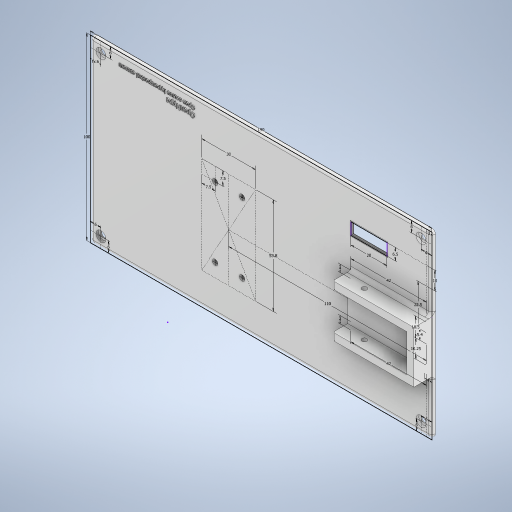
# Autodesk Inventor part: BoxCover
Saved by Autodesk Inventor 2023 (Build 270158000, 158)
## iProperties
Created: 2022-10-22
Part Number: BoxCover
Material: ABS Plastic
Document SubType Name: Modeling
Designer: Miner
Density: 1.06 g/cm^3
Appearance: Smooth - White
Author: Miner
Autodesk Inventor part; units mm, degrees
(part 1 of 2)
ref_plane "YZ Plane" through (0, 0, 0) normal (1, 0, 0) x (0, 1, 0)
ref_plane "XZ Plane" through (0, 0, 0) normal (0, 1, 0) x (-1, 0, 0)
ref_plane "XY Plane" through (0, 0, 0) normal (0, 0, 1) x (1, 0, 0)
sketch "Sketch1" plane through (0, 0, 0) normal (0, 0, 1) x (1, 0, 0)
  line L0 (0, 0) -> (-190, 0)
  line L1 (-190, 0) -> (-190, 100)
  line L2 (-190, 100) -> (0, 100)
  line L3 (0, 100) -> (0, 0)
  line L4 (0, 100) -> (-3, 100) construction
  line L5 (-3, 100) -> (-3, 0) construction
  line L6 (-3, 50) -> (-3, 44.6) construction
  line L7 (-3, 44.6) -> (-37.3438, 44.6) construction
  line L8 (-3, 44.6) -> (-3, 34.35) construction
  line L9 (-3, 34.35) -> (-45, 34.35)
  line L10 (-45, 34.35) -> (-45, 30.35)
  line L11 (-45, 30.35) -> (-3, 30.35)
  line L12 (-3, 30.35) -> (-3, 34.35)
  line L13 (-3, 44.6) -> (-3, 55.1) construction
  line L14 (-3, 55.1) -> (-45, 55.1)
  line L15 (-45, 55.1) -> (-45, 59.1)
  line L16 (-45, 59.1) -> (-3, 59.1)
  line L17 (-3, 59.1) -> (-3, 55.1)
  line L18 (0, 59.1) -> (-4, 59.1)
  line L19 (-4, 59.1) -> (-4, 30.35)
  line L20 (-4, 30.35) -> (0, 30.35)
  line L21 (0, 30.35) -> (0, 59.1)
  line L22 (-3, 44.6) -> (-113, 44.6) construction
  line L23 (-128, 17.7) -> (-98, 17.7) construction
  line L24 (-98, 17.7) -> (-98, 71.5) construction
  line L25 (-98, 71.5) -> (-128, 71.5) construction
  line L26 (-128, 71.5) -> (-128, 17.7) construction
  line L27 (-128, 17.7) -> (-98, 71.5) construction
  line L28 (-98, 17.7) -> (-128, 71.5) construction
  line L29 (-128, 71.5) -> (-120.5, 71.5) construction
  line L30 (-120.5, 71.5) -> (-120.5, 64) construction
  line L31 (-120.5, 64) -> (-128, 64) construction
  line L32 (-128, 64) -> (-128, 71.5) construction
  line L33 (-113, 71.5) -> (-113, 17.7) construction
  line L34 (-190, 100) -> (-184, 100) construction
  line L35 (-184, 100) -> (-184, 94) construction
  line L36 (-184, 94) -> (-190, 94) construction
  line L37 (-190, 94) -> (-190, 100) construction
  line L38 (0, 100) -> (-6, 100) construction
  line L39 (-6, 100) -> (-6, 94) construction
  line L40 (-6, 94) -> (0, 94) construction
  line L41 (0, 94) -> (0, 100) construction
  line L42 (0, 0) -> (-6, 0) construction
  line L43 (-6, 0) -> (-6, 6) construction
  line L44 (-6, 6) -> (0, 6) construction
  line L45 (0, 6) -> (0, 0) construction
  line L46 (-190, 0) -> (-184, 0) construction
  line L47 (-184, 0) -> (-184, 6) construction
  line L48 (-184, 6) -> (-190, 6) construction
  line L49 (-190, 6) -> (-190, 0) construction
  line L50 (-4, 55.1) -> (-45, 55.1)
  line L51 (-45, 55.1) -> (-45, 34.35)
  line L52 (-45, 34.35) -> (-4, 34.35)
  line L53 (-4, 34.35) -> (-4, 55.1)
  line L54 (-3, 50) -> (-3, 72.5) construction
  line L55 (-3, 72.5) -> (-3, 82.5) construction
  line L56 (-3, 82.5) -> (-45, 82.5) construction
  line L57 (-45, 82.5) -> (-25, 82.5) construction
  line L58 (-25, 82.5) -> (-25, 76)
  line L59 (-25, 76) -> (-45, 76)
  line L60 (-45, 76) -> (-45, 82.5)
  line L61 (-45, 82.5) -> (-25, 82.5)
  line L62 (-131.617, 88.8001) -> (-198.0641, 88.8001) construction
  line L63 (-198.0641, 88.8001) -> (-198.0641, 103.0152) construction
  line L64 (-198.0641, 103.0152) -> (-131.617, 103.0152) construction
  line L65 (-131.617, 103.0152) -> (-131.617, 88.8001) construction
  spline S0 degree 2 poles (-133.6389, 89.1384) (-133.7807, 89.3045) (-133.9387, 89.7908) (-133.9387, 90.1028) knots 0 0 0 1 2 2 2
  spline S1 degree 2 poles (-133.9387, 90.1028) (-133.9387, 90.4066) (-133.7847, 90.899) (-133.6389, 91.0651) knots 0 0 0 1 2 2 2
  spline S2 degree 2 poles (-133.6389, 91.0651) (-133.4849, 91.2393) (-133.0777, 91.4054) (-132.8326, 91.4054) knots 0 0 0 1 2 2 2
  spline S3 degree 2 poles (-132.8326, 91.4054) (-132.5793, 91.4054) (-132.1741, 91.2332) (-132.0262, 91.0651) knots 0 0 0 1 2 2 2
  spline S4 degree 2 poles (-132.0262, 91.0651) (-131.8824, 90.899) (-131.7284, 90.4107) (-131.7284, 90.1028) knots 0 0 0 1 2 2 2
  spline S5 degree 2 poles (-131.7284, 90.1028) (-131.7284, 89.7887) (-131.8844, 89.3106) (-132.0283, 89.1384) knots 0 0 0 1 2 2 2
  spline S6 degree 2 poles (-132.0283, 89.1384) (-132.1741, 88.9723) (-132.5813, 88.8001) (-132.8326, 88.8001) knots 0 0 0 1 2 2 2
  spline S7 degree 2 poles (-132.8326, 88.8001) (-133.0878, 88.8001) (-133.4971, 88.9784) (-133.6389, 89.1384) knots 0 0 0 1 2 2 2
  spline S8 degree 2 poles (-133.5923, 90.1028) (-133.5923, 89.8556) (-133.4849, 89.4727) (-133.3877, 89.3471) knots 0 0 0 1 2 2 2
  spline S9 degree 2 poles (-133.3877, 89.3471) (-133.2884, 89.2174) (-133.0088, 89.0878) (-132.8346, 89.0878) knots 0 0 0 1 2 2 2
  spline S10 degree 2 poles (-132.8346, 89.0878) (-132.6543, 89.0878) (-132.3828, 89.2134) (-132.2795, 89.3471) knots 0 0 0 1 2 2 2
  spline S11 degree 2 poles (-132.2795, 89.3471) (-132.1802, 89.4747) (-132.0749, 89.8596) (-132.0749, 90.1028) knots 0 0 0 1 2 2 2
  spline S12 degree 2 poles (-132.0749, 90.1028) (-132.0749, 90.5951) (-132.4881, 91.1178) (-132.8346, 91.1178) knots 0 0 0 1 2 2 2
  spline S13 degree 2 poles (-132.8346, 91.1178) (-133.181, 91.1178) (-133.5923, 90.5951) (-133.5923, 90.1028) knots 0 0 0 1 2 2 2
  spline S14 degree 2 poles (-135.8512, 90.3641) (-135.8512, 90.8341) (-135.4035, 91.3892) (-135.0611, 91.3892) knots 0 0 0 1 2 2 2
  spline S15 degree 2 poles (-135.0611, 91.3892) (-134.9213, 91.3892) (-134.7065, 91.3244) (-134.5951, 91.2575) knots 0 0 0 1 2 2 2
  line L66 (-134.5951, 91.2575) -> (-134.5951, 92.0436)
  line L67 (-134.5951, 92.0436) -> (-134.2791, 92.0436)
  line L68 (-134.2791, 92.0436) -> (-134.2791, 89.4767)
  line L69 (-134.2791, 89.4767) -> (-134.5951, 89.4767)
  line L70 (-134.5951, 89.4767) -> (-134.5951, 89.6733)
  spline S16 degree 2 poles (-134.5951, 89.6733) (-134.7126, 89.5659) (-135.0003, 89.4241) (-135.1685, 89.4241) knots 0 0 0 1 2 2 2
  spline S17 degree 2 poles (-135.1685, 89.4241) (-135.4906, 89.4241) (-135.8512, 89.9346) (-135.8512, 90.3641) knots 0 0 0 1 2 2 2
  spline S18 degree 2 poles (-135.525, 90.4006) (-135.525, 90.0784) (-135.3204, 89.7239) (-135.0915, 89.7239) knots 0 0 0 1 2 2 2
  spline S19 degree 2 poles (-135.0915, 89.7239) (-134.9578, 89.7239) (-134.7065, 89.8434) (-134.5951, 89.9366) knots 0 0 0 1 2 2 2
  line L71 (-134.5951, 89.9366) -> (-134.5951, 91.0023)
  spline S20 degree 2 poles (-134.5951, 91.0023) (-134.7187, 91.061) (-134.895, 91.1056) (-135.0084, 91.1056) knots 0 0 0 1 2 2 2
  spline S21 degree 2 poles (-135.0084, 91.1056) (-135.2535, 91.1056) (-135.525, 90.745) (-135.525, 90.4006) knots 0 0 0 1 2 2 2
  spline S22 degree 2 poles (-136.9938, 91.3953) (-136.5441, 91.3953) (-136.0497, 90.8908) (-136.0497, 90.4249) knots 0 0 0 1 2 2 2
  spline S23 degree 2 poles (-136.0497, 90.4249) (-136.0497, 89.967) (-136.5299, 89.4241) (-136.9168, 89.4241) knots 0 0 0 1 2 2 2
  spline S24 degree 2 poles (-136.9168, 89.4241) (-137.0911, 89.4241) (-137.3605, 89.5254) (-137.4598, 89.6327) knots 0 0 0 1 2 2 2
  spline S25 degree 2 poles (-137.4598, 89.6327) (-137.5611, 89.7401) (-137.6685, 90.0501) (-137.6685, 90.275) knots 0 0 0 1 2 2 2
  line L72 (-137.6685, 90.275) -> (-137.6685, 90.4472)
  line L73 (-137.6685, 90.4472) -> (-136.3698, 90.4472)
  spline S26 degree 2 poles (-136.3698, 90.4472) (-136.3698, 90.7733) (-136.698, 91.1198) (-136.9898, 91.1198) knots 0 0 0 1 2 2 2
  spline S27 degree 2 poles (-136.9898, 91.1198) (-137.0931, 91.1198) (-137.2937, 91.0732) (-137.3747, 91.0367) knots 0 0 0 1 2 2 2
  spline S28 degree 2 poles (-137.3747, 91.0367) (-137.4598, 90.9962) (-137.5773, 90.9253) (-137.6158, 90.8929) knots 0 0 0 1 2 2 2
  line L74 (-137.6158, 90.8929) -> (-137.634, 90.8929)
  line L75 (-137.634, 90.8929) -> (-137.634, 91.2373)
  spline S29 degree 2 poles (-137.634, 91.2373) (-137.5793, 91.2596) (-137.4132, 91.3244) (-137.3484, 91.3426) knots 0 0 0 1 2 2 2
  spline S30 degree 2 poles (-137.3484, 91.3426) (-137.2572, 91.369) (-137.1073, 91.3953) (-136.9938, 91.3953) knots 0 0 0 1 2 2 2
  spline S31 degree 2 poles (-137.3605, 90.2061) (-137.3565, 90.0784) (-137.3038, 89.8921) (-137.2531, 89.8293) knots 0 0 0 1 2 2 2
  spline S32 degree 2 poles (-137.2531, 89.8293) (-137.1984, 89.7584) (-137.0262, 89.6834) (-136.8986, 89.6834) knots 0 0 0 1 2 2 2
  spline S33 degree 2 poles (-136.8986, 89.6834) (-136.773, 89.6834) (-136.5967, 89.7584) (-136.5238, 89.8313) knots 0 0 0 1 2 2 2
  spline S34 degree 2 poles (-136.5238, 89.8313) (-136.4529, 89.9062) (-136.38, 90.0866) (-136.3698, 90.2061) knots 0 0 0 1 2 2 2
  line L76 (-136.3698, 90.2061) -> (-137.3605, 90.2061)
  line L77 (-139.4614, 91.3528) -> (-139.1454, 91.3528)
  line L78 (-139.1454, 91.3528) -> (-139.1454, 90.2831)
  spline S35 degree 2 poles (-139.1454, 90.2831) (-139.1454, 90.1534) (-139.121, 89.9306) (-139.0846, 89.8637) knots 0 0 0 1 2 2 2
  spline S36 degree 2 poles (-139.0846, 89.8637) (-139.0461, 89.7928) (-138.9083, 89.7239) (-138.7908, 89.7239) knots 0 0 0 1 2 2 2
  spline S37 degree 2 poles (-138.7908, 89.7239) (-138.6733, 89.7239) (-138.4241, 89.8495) (-138.3046, 89.9508) knots 0 0 0 1 2 2 2
  line L79 (-138.3046, 89.9508) -> (-138.3046, 91.3528)
  line L80 (-138.3046, 91.3528) -> (-137.9885, 91.3528)
  line L81 (-137.9885, 91.3528) -> (-137.9885, 89.4767)
  line L82 (-137.9885, 89.4767) -> (-138.3046, 89.4767)
  line L83 (-138.3046, 89.4767) -> (-138.3046, 89.6854)
  spline S38 degree 2 poles (-138.3046, 89.6854) (-138.4464, 89.5578) (-138.7199, 89.4241) (-138.8739, 89.4241) knots 0 0 0 1 2 2 2
  spline S39 degree 2 poles (-138.8739, 89.4241) (-139.1494, 89.4241) (-139.4614, 89.7887) (-139.4614, 90.1352) knots 0 0 0 1 2 2 2
  line L84 (-139.4614, 90.1352) -> (-139.4614, 91.3528)
  line L85 (-141.7446, 91.3528) -> (-141.4124, 91.3528)
  line L86 (-141.4124, 91.3528) -> (-141.4124, 90.1291)
  line L87 (-141.4124, 90.1291) -> (-140.2616, 90.1291)
  line L88 (-140.2616, 90.1291) -> (-140.2616, 91.3528)
  line L89 (-140.2616, 91.3528) -> (-139.9294, 91.3528)
  line L90 (-139.9294, 91.3528) -> (-139.9294, 88.8528)
  line L91 (-139.9294, 88.8528) -> (-140.2616, 88.8528)
  line L92 (-140.2616, 88.8528) -> (-140.2616, 89.8333)
  line L93 (-140.2616, 89.8333) -> (-141.4124, 89.8333)
  line L94 (-141.4124, 89.8333) -> (-141.4124, 88.8528)
  line L95 (-141.4124, 88.8528) -> (-141.7446, 88.8528)
  line L96 (-141.7446, 88.8528) -> (-141.7446, 91.3528)
  line L97 (-143.6997, 89.4767) -> (-142.6907, 92.0436)
  line L98 (-142.6907, 92.0436) -> (-142.3524, 92.0436)
  line L99 (-142.3524, 92.0436) -> (-142.6887, 91.2616)
  line L100 (-142.6887, 91.2616) -> (-142.008, 89.4767)
  line L101 (-142.008, 89.4767) -> (-142.3484, 89.4767)
  line L102 (-142.3484, 89.4767) -> (-142.8609, 90.8665)
  line L103 (-142.8609, 90.8665) -> (-143.3714, 89.4767)
  line L104 (-143.3714, 89.4767) -> (-143.6997, 89.4767)
  spline S40 degree 2 poles (-145.5108, 90.3641) (-145.5108, 90.8341) (-145.0631, 91.3892) (-144.7207, 91.3892) knots 0 0 0 1 2 2 2
  spline S41 degree 2 poles (-144.7207, 91.3892) (-144.5809, 91.3892) (-144.3662, 91.3244) (-144.2548, 91.2575) knots 0 0 0 1 2 2 2
  line L105 (-144.2548, 91.2575) -> (-144.2548, 92.0436)
  line L106 (-144.2548, 92.0436) -> (-143.9387, 92.0436)
  line L107 (-143.9387, 92.0436) -> (-143.9387, 89.4767)
  line L108 (-143.9387, 89.4767) -> (-144.2548, 89.4767)
  line L109 (-144.2548, 89.4767) -> (-144.2548, 89.6733)
  spline S42 degree 2 poles (-144.2548, 89.6733) (-144.3723, 89.5659) (-144.6599, 89.4241) (-144.8281, 89.4241) knots 0 0 0 1 2 2 2
  spline S43 degree 2 poles (-144.8281, 89.4241) (-145.1502, 89.4241) (-145.5108, 89.9346) (-145.5108, 90.3641) knots 0 0 0 1 2 2 2
  spline S44 degree 2 poles (-145.1847, 90.4006) (-145.1847, 90.0784) (-144.98, 89.7239) (-144.7511, 89.7239) knots 0 0 0 1 2 2 2
  spline S45 degree 2 poles (-144.7511, 89.7239) (-144.6174, 89.7239) (-144.3662, 89.8434) (-144.2548, 89.9366) knots 0 0 0 1 2 2 2
  line L110 (-144.2548, 89.9366) -> (-144.2548, 91.0023)
  spline S46 degree 2 poles (-144.2548, 91.0023) (-144.3783, 91.061) (-144.5546, 91.1056) (-144.668, 91.1056) knots 0 0 0 1 2 2 2
  spline S47 degree 2 poles (-144.668, 91.1056) (-144.9132, 91.1056) (-145.1847, 90.745) (-145.1847, 90.4006) knots 0 0 0 1 2 2 2
  spline S48 degree 2 poles (-146.6535, 91.3953) (-146.2037, 91.3953) (-145.7094, 90.8908) (-145.7094, 90.4249) knots 0 0 0 1 2 2 2
  spline S49 degree 2 poles (-145.7094, 90.4249) (-145.7094, 89.967) (-146.1895, 89.4241) (-146.5765, 89.4241) knots 0 0 0 1 2 2 2
  spline S50 degree 2 poles (-146.5765, 89.4241) (-146.7507, 89.4241) (-147.0202, 89.5254) (-147.1194, 89.6327) knots 0 0 0 1 2 2 2
  spline S51 degree 2 poles (-147.1194, 89.6327) (-147.2207, 89.7401) (-147.3281, 90.0501) (-147.3281, 90.275) knots 0 0 0 1 2 2 2
  line L111 (-147.3281, 90.275) -> (-147.3281, 90.4472)
  line L112 (-147.3281, 90.4472) -> (-146.0295, 90.4472)
  spline S52 degree 2 poles (-146.0295, 90.4472) (-146.0295, 90.7733) (-146.3577, 91.1198) (-146.6494, 91.1198) knots 0 0 0 1 2 2 2
  spline S53 degree 2 poles (-146.6494, 91.1198) (-146.7527, 91.1198) (-146.9533, 91.0732) (-147.0343, 91.0367) knots 0 0 0 1 2 2 2
  spline S54 degree 2 poles (-147.0343, 91.0367) (-147.1194, 90.9962) (-147.2369, 90.9253) (-147.2754, 90.8929) knots 0 0 0 1 2 2 2
  line L113 (-147.2754, 90.8929) -> (-147.2937, 90.8929)
  line L114 (-147.2937, 90.8929) -> (-147.2937, 91.2373)
  spline S55 degree 2 poles (-147.2937, 91.2373) (-147.239, 91.2596) (-147.0728, 91.3244) (-147.008, 91.3426) knots 0 0 0 1 2 2 2
  spline S56 degree 2 poles (-147.008, 91.3426) (-146.9168, 91.369) (-146.7669, 91.3953) (-146.6535, 91.3953) knots 0 0 0 1 2 2 2
  spline S57 degree 2 poles (-147.0202, 90.2061) (-147.0161, 90.0784) (-146.9634, 89.8921) (-146.9128, 89.8293) knots 0 0 0 1 2 2 2
  spline S58 degree 2 poles (-146.9128, 89.8293) (-146.8581, 89.7584) (-146.6859, 89.6834) (-146.5582, 89.6834) knots 0 0 0 1 2 2 2
  spline S59 degree 2 poles (-146.5582, 89.6834) (-146.4326, 89.6834) (-146.2564, 89.7584) (-146.1834, 89.8313) knots 0 0 0 1 2 2 2
  spline S60 degree 2 poles (-146.1834, 89.8313) (-146.1125, 89.9062) (-146.0396, 90.0866) (-146.0295, 90.2061) knots 0 0 0 1 2 2 2
  line L115 (-146.0295, 90.2061) -> (-147.0202, 90.2061)
  spline S61 degree 2 poles (-133.2345, 93.0672) (-133.3479, 93.2001) (-133.4744, 93.5891) (-133.4744, 93.8387) knots 0 0 0 1 2 2 2
  spline S62 degree 2 poles (-133.4744, 93.8387) (-133.4744, 94.0818) (-133.3512, 94.4756) (-133.2345, 94.6085) knots 0 0 0 1 2 2 2
  spline S63 degree 2 poles (-133.2345, 94.6085) (-133.1113, 94.7479) (-132.7856, 94.8808) (-132.5894, 94.8808) knots 0 0 0 1 2 2 2
  spline S64 degree 2 poles (-132.5894, 94.8808) (-132.3868, 94.8808) (-132.0627, 94.743) (-131.9444, 94.6085) knots 0 0 0 1 2 2 2
  spline S65 degree 2 poles (-131.9444, 94.6085) (-131.8293, 94.4756) (-131.7061, 94.085) (-131.7061, 93.8387) knots 0 0 0 1 2 2 2
  spline S66 degree 2 poles (-131.7061, 93.8387) (-131.7061, 93.5874) (-131.8309, 93.2049) (-131.946, 93.0672) knots 0 0 0 1 2 2 2
  spline S67 degree 2 poles (-131.946, 93.0672) (-132.0627, 92.9343) (-132.3885, 92.7965) (-132.5894, 92.7965) knots 0 0 0 1 2 2 2
  spline S68 degree 2 poles (-132.5894, 92.7965) (-132.7937, 92.7965) (-133.121, 92.9391) (-133.2345, 93.0672) knots 0 0 0 1 2 2 2
  spline S69 degree 2 poles (-133.1972, 93.8387) (-133.1972, 93.6409) (-133.1113, 93.3346) (-133.0335, 93.2341) knots 0 0 0 1 2 2 2
  spline S70 degree 2 poles (-133.0335, 93.2341) (-132.9541, 93.1304) (-132.7304, 93.0267) (-132.5911, 93.0267) knots 0 0 0 1 2 2 2
  spline S71 degree 2 poles (-132.5911, 93.0267) (-132.4468, 93.0267) (-132.2296, 93.1271) (-132.147, 93.2341) knots 0 0 0 1 2 2 2
  spline S72 degree 2 poles (-132.147, 93.2341) (-132.0676, 93.3362) (-131.9833, 93.6442) (-131.9833, 93.8387) knots 0 0 0 1 2 2 2
  spline S73 degree 2 poles (-131.9833, 93.8387) (-131.9833, 94.2325) (-132.3139, 94.6506) (-132.5911, 94.6506) knots 0 0 0 1 2 2 2
  spline S74 degree 2 poles (-132.5911, 94.6506) (-132.8682, 94.6506) (-133.1972, 94.2325) (-133.1972, 93.8387) knots 0 0 0 1 2 2 2
  spline S75 degree 2 poles (-135.0044, 94.0477) (-135.0044, 94.4237) (-134.6462, 94.8678) (-134.3723, 94.8678) knots 0 0 0 1 2 2 2
  spline S76 degree 2 poles (-134.3723, 94.8678) (-134.2604, 94.8678) (-134.0886, 94.816) (-133.9995, 94.7625) knots 0 0 0 1 2 2 2
  line L116 (-133.9995, 94.7625) -> (-133.9995, 95.3913)
  line L117 (-133.9995, 95.3913) -> (-133.7467, 95.3913)
  line L118 (-133.7467, 95.3913) -> (-133.7467, 93.3378)
  line L119 (-133.7467, 93.3378) -> (-133.9995, 93.3378)
  line L120 (-133.9995, 93.3378) -> (-133.9995, 93.4951)
  spline S77 degree 2 poles (-133.9995, 93.4951) (-134.0935, 93.4092) (-134.3236, 93.2957) (-134.4582, 93.2957) knots 0 0 0 1 2 2 2
  spline S78 degree 2 poles (-134.4582, 93.2957) (-134.7159, 93.2957) (-135.0044, 93.7041) (-135.0044, 94.0477) knots 0 0 0 1 2 2 2
  spline S79 degree 2 poles (-134.7434, 94.0769) (-134.7434, 93.8192) (-134.5797, 93.5356) (-134.3966, 93.5356) knots 0 0 0 1 2 2 2
  spline S80 degree 2 poles (-134.3966, 93.5356) (-134.2896, 93.5356) (-134.0886, 93.6312) (-133.9995, 93.7058) knots 0 0 0 1 2 2 2
  line L121 (-133.9995, 93.7058) -> (-133.9995, 94.5583)
  spline S81 degree 2 poles (-133.9995, 94.5583) (-134.0984, 94.6053) (-134.2394, 94.6409) (-134.3301, 94.6409) knots 0 0 0 1 2 2 2
  spline S82 degree 2 poles (-134.3301, 94.6409) (-134.5262, 94.6409) (-134.7434, 94.3524) (-134.7434, 94.0769) knots 0 0 0 1 2 2 2
  spline S83 degree 2 poles (-135.9185, 94.8727) (-135.5586, 94.8727) (-135.1632, 94.4691) (-135.1632, 94.0964) knots 0 0 0 1 2 2 2
  spline S84 degree 2 poles (-135.1632, 94.0964) (-135.1632, 93.7301) (-135.5473, 93.2957) (-135.8569, 93.2957) knots 0 0 0 1 2 2 2
  spline S85 degree 2 poles (-135.8569, 93.2957) (-135.9962, 93.2957) (-136.2118, 93.3767) (-136.2912, 93.4626) knots 0 0 0 1 2 2 2
  spline S86 degree 2 poles (-136.2912, 93.4626) (-136.3723, 93.5485) (-136.4582, 93.7965) (-136.4582, 93.9764) knots 0 0 0 1 2 2 2
  line L122 (-136.4582, 93.9764) -> (-136.4582, 94.1142)
  line L123 (-136.4582, 94.1142) -> (-135.4193, 94.1142)
  spline S87 degree 2 poles (-135.4193, 94.1142) (-135.4193, 94.3751) (-135.6818, 94.6523) (-135.9152, 94.6523) knots 0 0 0 1 2 2 2
  spline S88 degree 2 poles (-135.9152, 94.6523) (-135.9979, 94.6523) (-136.1583, 94.615) (-136.2232, 94.5858) knots 0 0 0 1 2 2 2
  spline S89 degree 2 poles (-136.2232, 94.5858) (-136.2912, 94.5534) (-136.3852, 94.4967) (-136.416, 94.4707) knots 0 0 0 1 2 2 2
  line L124 (-136.416, 94.4707) -> (-136.4306, 94.4707)
  line L125 (-136.4306, 94.4707) -> (-136.4306, 94.7463)
  spline S90 degree 2 poles (-136.4306, 94.7463) (-136.3868, 94.7641) (-136.2539, 94.816) (-136.2021, 94.8306) knots 0 0 0 1 2 2 2
  spline S91 degree 2 poles (-136.2021, 94.8306) (-136.1291, 94.8516) (-136.0092, 94.8727) (-135.9185, 94.8727) knots 0 0 0 1 2 2 2
  spline S92 degree 2 poles (-136.2118, 93.9213) (-136.2086, 93.8192) (-136.1664, 93.6701) (-136.1259, 93.6199) knots 0 0 0 1 2 2 2
  spline S93 degree 2 poles (-136.1259, 93.6199) (-136.0821, 93.5631) (-135.9444, 93.5032) (-135.8423, 93.5032) knots 0 0 0 1 2 2 2
  spline S94 degree 2 poles (-135.8423, 93.5032) (-135.7418, 93.5032) (-135.6008, 93.5631) (-135.5424, 93.6215) knots 0 0 0 1 2 2 2
  spline S95 degree 2 poles (-135.5424, 93.6215) (-135.4857, 93.6814) (-135.4274, 93.8257) (-135.4193, 93.9213) knots 0 0 0 1 2 2 2
  line L126 (-135.4193, 93.9213) -> (-136.2118, 93.9213)
  line L127 (-137.8925, 94.8387) -> (-137.6397, 94.8387)
  line L128 (-137.6397, 94.8387) -> (-137.6397, 93.9829)
  spline S96 degree 2 poles (-137.6397, 93.9829) (-137.6397, 93.8792) (-137.6202, 93.7009) (-137.5911, 93.6474) knots 0 0 0 1 2 2 2
  spline S97 degree 2 poles (-137.5911, 93.6474) (-137.5603, 93.5907) (-137.4501, 93.5356) (-137.3561, 93.5356) knots 0 0 0 1 2 2 2
  spline S98 degree 2 poles (-137.3561, 93.5356) (-137.262, 93.5356) (-137.0627, 93.6361) (-136.9671, 93.7171) knots 0 0 0 1 2 2 2
  line L129 (-136.9671, 93.7171) -> (-136.9671, 94.8387)
  line L130 (-136.9671, 94.8387) -> (-136.7142, 94.8387)
  line L131 (-136.7142, 94.8387) -> (-136.7142, 93.3378)
  line L132 (-136.7142, 93.3378) -> (-136.9671, 93.3378)
  line L133 (-136.9671, 93.3378) -> (-136.9671, 93.5048)
  spline S99 degree 2 poles (-136.9671, 93.5048) (-137.0805, 93.4027) (-137.2993, 93.2957) (-137.4225, 93.2957) knots 0 0 0 1 2 2 2
  spline S100 degree 2 poles (-137.4225, 93.2957) (-137.6429, 93.2957) (-137.8925, 93.5874) (-137.8925, 93.8646) knots 0 0 0 1 2 2 2
  line L134 (-137.8925, 93.8646) -> (-137.8925, 94.8387)
  spline S101 degree 2 poles (-139.5116, 94.8743) (-139.3609, 94.8743) (-139.1, 94.7933) (-139.0141, 94.7479) knots 0 0 0 1 2 2 2
  line L135 (-139.0141, 94.7479) -> (-139.0141, 94.4643)
  line L136 (-139.0141, 94.4643) -> (-139.027, 94.4643)
  spline S102 degree 2 poles (-139.027, 94.4643) (-139.0595, 94.4902) (-139.147, 94.5518) (-139.2199, 94.5858) knots 0 0 0 1 2 2 2
  spline S103 degree 2 poles (-139.2199, 94.5858) (-139.2831, 94.6166) (-139.4387, 94.662) (-139.5214, 94.662) knots 0 0 0 1 2 2 2
  spline S104 degree 2 poles (-139.5214, 94.662) (-139.5813, 94.662) (-139.7191, 94.6344) (-139.7515, 94.6118) knots 0 0 0 1 2 2 2
  spline S105 degree 2 poles (-139.7515, 94.6118) (-139.7985, 94.581) (-139.8407, 94.5113) (-139.8407, 94.44) knots 0 0 0 1 2 2 2
  spline S106 degree 2 poles (-139.8407, 94.44) (-139.8407, 94.3508) (-139.7434, 94.2584) (-139.6186, 94.2276) knots 0 0 0 1 2 2 2
  spline S107 degree 2 poles (-139.6186, 94.2276) (-139.57, 94.2163) (-139.4144, 94.1839) (-139.3479, 94.166) knots 0 0 0 1 2 2 2
  spline S108 degree 2 poles (-139.3479, 94.166) (-139.1762, 94.1158) (-139.0206, 93.9083) (-139.0206, 93.7609) knots 0 0 0 1 2 2 2
  spline S109 degree 2 poles (-139.0206, 93.7609) (-139.0206, 93.5566) (-139.3269, 93.3022) (-139.5797, 93.3022) knots 0 0 0 1 2 2 2
  spline S110 degree 2 poles (-139.5797, 93.3022) (-139.7045, 93.3022) (-139.9573, 93.3638) (-140.0432, 93.4108) knots 0 0 0 1 2 2 2
  line L137 (-140.0432, 93.4108) -> (-140.0432, 93.6814)
  line L138 (-140.0432, 93.6814) -> (-140.0303, 93.6814)
  spline S111 degree 2 poles (-140.0303, 93.6814) (-139.933, 93.6036) (-139.6964, 93.5145) (-139.5749, 93.5145) knots 0 0 0 1 2 2 2
  spline S112 degree 2 poles (-139.5749, 93.5145) (-139.4501, 93.5145) (-139.2783, 93.6199) (-139.2783, 93.7252) knots 0 0 0 1 2 2 2
  spline S113 degree 2 poles (-139.2783, 93.7252) (-139.2783, 93.8208) (-139.3804, 93.9132) (-139.4938, 93.9424) knots 0 0 0 1 2 2 2
  spline S114 degree 2 poles (-139.4938, 93.9424) (-139.5489, 93.957) (-139.6883, 93.9861) (-139.7645, 94.004) knots 0 0 0 1 2 2 2
  spline S115 degree 2 poles (-139.7645, 94.004) (-139.9298, 94.0461) (-140.0984, 94.239) (-140.0984, 94.4059) knots 0 0 0 1 2 2 2
  spline S116 degree 2 poles (-140.0984, 94.4059) (-140.0984, 94.5032) (-140.0222, 94.675) (-139.9476, 94.7382) knots 0 0 0 1 2 2 2
  spline S117 degree 2 poles (-139.9476, 94.7382) (-139.8682, 94.8046) (-139.6656, 94.8743) (-139.5116, 94.8743) knots 0 0 0 1 2 2 2
  spline S118 degree 2 poles (-141.5667, 94.0882) (-141.5667, 94.4675) (-141.2021, 94.8808) (-140.8974, 94.8808) knots 0 0 0 1 2 2 2
  spline S119 degree 2 poles (-140.8974, 94.8808) (-140.5846, 94.8808) (-140.2264, 94.4545) (-140.2264, 94.0882) knots 0 0 0 1 2 2 2
  spline S120 degree 2 poles (-140.2264, 94.0882) (-140.2264, 93.7122) (-140.5959, 93.2957) (-140.8974, 93.2957) knots 0 0 0 1 2 2 2
  spline S121 degree 2 poles (-140.8974, 93.2957) (-141.2021, 93.2957) (-141.5667, 93.7106) (-141.5667, 94.0882) knots 0 0 0 1 2 2 2
  spline S122 degree 2 poles (-141.3058, 94.0882) (-141.3058, 93.7965) (-141.0935, 93.5129) (-140.8974, 93.5129) knots 0 0 0 1 2 2 2
  spline S123 degree 2 poles (-140.8974, 93.5129) (-140.7013, 93.5129) (-140.4873, 93.7965) (-140.4873, 94.0882) knots 0 0 0 1 2 2 2
  spline S124 degree 2 poles (-140.4873, 94.0882) (-140.4873, 94.3719) (-140.7013, 94.6636) (-140.8974, 94.6636) knots 0 0 0 1 2 2 2
  spline S125 degree 2 poles (-140.8974, 94.6636) (-141.0919, 94.6636) (-141.3058, 94.3767) (-141.3058, 94.0882) knots 0 0 0 1 2 2 2
  line L139 (-142.993, 94.8387) -> (-142.7402, 94.8387)
  line L140 (-142.7402, 94.8387) -> (-142.7402, 94.6733)
  spline S126 degree 2 poles (-142.7402, 94.6733) (-142.6235, 94.7754) (-142.4144, 94.8808) (-142.2847, 94.8808) knots 0 0 0 1 2 2 2
  spline S127 degree 2 poles (-142.2847, 94.8808) (-142.1875, 94.8808) (-142.0141, 94.816) (-141.9509, 94.7463) knots 0 0 0 1 2 2 2
  spline S128 degree 2 poles (-141.9509, 94.7463) (-141.886, 94.6766) (-141.8147, 94.4643) (-141.8147, 94.3119) knots 0 0 0 1 2 2 2
  line L141 (-141.8147, 94.3119) -> (-141.8147, 93.3378)
  line L142 (-141.8147, 93.3378) -> (-142.0676, 93.3378)
  line L143 (-142.0676, 93.3378) -> (-142.0676, 94.1936)
  spline S129 degree 2 poles (-142.0676, 94.1936) (-142.0676, 94.3135) (-142.0854, 94.4707) (-142.1162, 94.5291) knots 0 0 0 1 2 2 2
  spline S130 degree 2 poles (-142.1162, 94.5291) (-142.147, 94.5874) (-142.2523, 94.6409) (-142.3512, 94.6409) knots 0 0 0 1 2 2 2
  spline S131 degree 2 poles (-142.3512, 94.6409) (-142.4436, 94.6409) (-142.6526, 94.5356) (-142.7402, 94.4594) knots 0 0 0 1 2 2 2
  line L144 (-142.7402, 94.4594) -> (-142.7402, 93.3378)
  line L145 (-142.7402, 93.3378) -> (-142.993, 93.3378)
  line L146 (-142.993, 93.3378) -> (-142.993, 94.8387)
  line L147 (-144.1551, 93.6085) -> (-144.1421, 93.6085)
  spline S132 degree 2 poles (-144.1421, 93.6085) (-144.1129, 93.6004) (-144.0497, 93.5972) (-144.006, 93.5972) knots 0 0 0 1 2 2 2
  spline S133 degree 2 poles (-144.006, 93.5972) (-143.9039, 93.5972) (-143.7029, 93.6863) (-143.6121, 93.7738) knots 0 0 0 1 2 2 2
  line L148 (-143.6121, 93.7738) -> (-143.6121, 94.8387)
  line L149 (-143.6121, 94.8387) -> (-143.3593, 94.8387)
  line L150 (-143.3593, 94.8387) -> (-143.3593, 93.3378)
  line L151 (-143.3593, 93.3378) -> (-143.6121, 93.3378)
  line L152 (-143.6121, 93.3378) -> (-143.6121, 93.5615)
  spline S134 degree 2 poles (-143.6121, 93.5615) (-143.7499, 93.4383) (-143.9557, 93.3378) (-144.053, 93.3378) knots 0 0 0 1 2 2 2
  spline S135 degree 2 poles (-144.053, 93.3378) (-144.0919, 93.3378) (-144.1308, 93.3411) (-144.1551, 93.3459) knots 0 0 0 1 2 2 2
  line L153 (-144.1551, 93.3459) -> (-144.1551, 93.6085)
  spline S136 degree 2 poles (-144.9476, 94.8727) (-144.792, 94.8727) (-144.5343, 94.7771) (-144.442, 94.6798) knots 0 0 0 1 2 2 2
  spline S137 degree 2 poles (-144.442, 94.6798) (-144.3496, 94.5842) (-144.2475, 94.2892) (-144.2475, 94.0915) knots 0 0 0 1 2 2 2
  spline S138 degree 2 poles (-144.2475, 94.0915) (-144.2475, 93.8938) (-144.3528, 93.6053) (-144.442, 93.508) knots 0 0 0 1 2 2 2
  spline S139 degree 2 poles (-144.442, 93.508) (-144.5311, 93.4092) (-144.7953, 93.3038) (-144.9476, 93.3038) knots 0 0 0 1 2 2 2
  spline S140 degree 2 poles (-144.9476, 93.3038) (-145.0708, 93.3038) (-145.3009, 93.3735) (-145.3901, 93.4189) knots 0 0 0 1 2 2 2
  line L154 (-145.3901, 93.4189) -> (-145.3901, 93.7025)
  line L155 (-145.3901, 93.7025) -> (-145.3755, 93.7025)
  spline S141 degree 2 poles (-145.3755, 93.7025) (-145.3479, 93.6798) (-145.2637, 93.6215) (-145.2037, 93.5907) knots 0 0 0 1 2 2 2
  spline S142 degree 2 poles (-145.2037, 93.5907) (-145.1502, 93.5647) (-145.0076, 93.5242) (-144.9428, 93.5242) knots 0 0 0 1 2 2 2
  spline S143 degree 2 poles (-144.9428, 93.5242) (-144.7467, 93.5242) (-144.5084, 93.8208) (-144.5084, 94.0915) knots 0 0 0 1 2 2 2
  spline S144 degree 2 poles (-144.5084, 94.0915) (-144.5084, 94.3557) (-144.7385, 94.6523) (-144.9428, 94.6523) knots 0 0 0 1 2 2 2
  spline S145 degree 2 poles (-144.9428, 94.6523) (-145.0659, 94.6523) (-145.2896, 94.5502) (-145.3755, 94.4707) knots 0 0 0 1 2 2 2
  line L156 (-145.3755, 94.4707) -> (-145.3901, 94.4707)
  line L157 (-145.3901, 94.4707) -> (-145.3901, 94.7544)
  spline S146 degree 2 poles (-145.3901, 94.7544) (-145.3528, 94.7722) (-145.2394, 94.8224) (-145.194, 94.8338) knots 0 0 0 1 2 2 2
  spline S147 degree 2 poles (-145.194, 94.8338) (-145.1291, 94.8532) (-145.027, 94.8727) (-144.9476, 94.8727) knots 0 0 0 1 2 2 2
  spline S148 degree 2 poles (-146.2718, 94.8727) (-145.912, 94.8727) (-145.5165, 94.4691) (-145.5165, 94.0964) knots 0 0 0 1 2 2 2
  spline S149 degree 2 poles (-145.5165, 94.0964) (-145.5165, 93.7301) (-145.9006, 93.2957) (-146.2102, 93.2957) knots 0 0 0 1 2 2 2
  spline S150 degree 2 poles (-146.2102, 93.2957) (-146.3496, 93.2957) (-146.5651, 93.3767) (-146.6445, 93.4626) knots 0 0 0 1 2 2 2
  spline S151 degree 2 poles (-146.6445, 93.4626) (-146.7256, 93.5485) (-146.8115, 93.7965) (-146.8115, 93.9764) knots 0 0 0 1 2 2 2
  line L158 (-146.8115, 93.9764) -> (-146.8115, 94.1142)
  line L159 (-146.8115, 94.1142) -> (-145.7726, 94.1142)
  spline S152 degree 2 poles (-145.7726, 94.1142) (-145.7726, 94.3751) (-146.0351, 94.6523) (-146.2685, 94.6523) knots 0 0 0 1 2 2 2
  spline S153 degree 2 poles (-146.2685, 94.6523) (-146.3512, 94.6523) (-146.5116, 94.615) (-146.5765, 94.5858) knots 0 0 0 1 2 2 2
  spline S154 degree 2 poles (-146.5765, 94.5858) (-146.6445, 94.5534) (-146.7385, 94.4967) (-146.7693, 94.4707) knots 0 0 0 1 2 2 2
  line L160 (-146.7693, 94.4707) -> (-146.7839, 94.4707)
  line L161 (-146.7839, 94.4707) -> (-146.7839, 94.7463)
  spline S155 degree 2 poles (-146.7839, 94.7463) (-146.7402, 94.7641) (-146.6073, 94.816) (-146.5554, 94.8306) knots 0 0 0 1 2 2 2
  spline S156 degree 2 poles (-146.5554, 94.8306) (-146.4825, 94.8516) (-146.3625, 94.8727) (-146.2718, 94.8727) knots 0 0 0 1 2 2 2
  spline S157 degree 2 poles (-146.5651, 93.9213) (-146.5619, 93.8192) (-146.5197, 93.6701) (-146.4792, 93.6199) knots 0 0 0 1 2 2 2
  spline S158 degree 2 poles (-146.4792, 93.6199) (-146.4355, 93.5631) (-146.2977, 93.5032) (-146.1956, 93.5032) knots 0 0 0 1 2 2 2
  spline S159 degree 2 poles (-146.1956, 93.5032) (-146.0951, 93.5032) (-145.9541, 93.5631) (-145.8958, 93.6215) knots 0 0 0 1 2 2 2
  spline S160 degree 2 poles (-145.8958, 93.6215) (-145.839, 93.6814) (-145.7807, 93.8257) (-145.7726, 93.9213) knots 0 0 0 1 2 2 2
  line L162 (-145.7726, 93.9213) -> (-146.5651, 93.9213)
  line L163 (-149.1048, 94.8387) -> (-148.852, 94.8387)
  line L164 (-148.852, 94.8387) -> (-148.852, 93.9829)
  spline S161 degree 2 poles (-148.852, 93.9829) (-148.852, 93.8792) (-148.8326, 93.7009) (-148.8034, 93.6474) knots 0 0 0 1 2 2 2
  spline S162 degree 2 poles (-148.8034, 93.6474) (-148.7726, 93.5907) (-148.6624, 93.5356) (-148.5684, 93.5356) knots 0 0 0 1 2 2 2
  spline S163 degree 2 poles (-148.5684, 93.5356) (-148.4744, 93.5356) (-148.275, 93.6361) (-148.1794, 93.7171) knots 0 0 0 1 2 2 2
  line L165 (-148.1794, 93.7171) -> (-148.1794, 94.8387)
  line L166 (-148.1794, 94.8387) -> (-147.9266, 94.8387)
  line L167 (-147.9266, 94.8387) -> (-147.9266, 92.7495)
  line L168 (-147.9266, 92.7495) -> (-148.1794, 92.7495)
  line L169 (-148.1794, 92.7495) -> (-148.1794, 93.5048)
  spline S164 degree 2 poles (-148.1794, 93.5048) (-148.2928, 93.4027) (-148.5116, 93.2957) (-148.6348, 93.2957) knots 0 0 0 1 2 2 2
  spline S165 degree 2 poles (-148.6348, 93.2957) (-148.8552, 93.2957) (-149.1048, 93.5874) (-149.1048, 93.8646) knots 0 0 0 1 2 2 2
  line L170 (-149.1048, 93.8646) -> (-149.1048, 94.8387)
  line L171 (-150.6381, 93.3378) -> (-149.8309, 95.3913)
  line L172 (-149.8309, 95.3913) -> (-149.5603, 95.3913)
  line L173 (-149.5603, 95.3913) -> (-149.8293, 94.7657)
  line L174 (-149.8293, 94.7657) -> (-149.2847, 93.3378)
  line L175 (-149.2847, 93.3378) -> (-149.557, 93.3378)
  line L176 (-149.557, 93.3378) -> (-149.9671, 94.4497)
  line L177 (-149.9671, 94.4497) -> (-150.3755, 93.3378)
  line L178 (-150.3755, 93.3378) -> (-150.6381, 93.3378)
  spline S166 degree 2 poles (-152.087, 94.0477) (-152.087, 94.4237) (-151.7288, 94.8678) (-151.4549, 94.8678) knots 0 0 0 1 2 2 2
  spline S167 degree 2 poles (-151.4549, 94.8678) (-151.3431, 94.8678) (-151.1713, 94.816) (-151.0821, 94.7625) knots 0 0 0 1 2 2 2
  line L179 (-151.0821, 94.7625) -> (-151.0821, 95.3913)
  line L180 (-151.0821, 95.3913) -> (-150.8293, 95.3913)
  line L181 (-150.8293, 95.3913) -> (-150.8293, 93.3378)
  line L182 (-150.8293, 93.3378) -> (-151.0821, 93.3378)
  line L183 (-151.0821, 93.3378) -> (-151.0821, 93.4951)
  spline S168 degree 2 poles (-151.0821, 93.4951) (-151.1762, 93.4092) (-151.4063, 93.2957) (-151.5408, 93.2957) knots 0 0 0 1 2 2 2
  spline S169 degree 2 poles (-151.5408, 93.2957) (-151.7985, 93.2957) (-152.087, 93.7041) (-152.087, 94.0477) knots 0 0 0 1 2 2 2
  spline S170 degree 2 poles (-151.8261, 94.0769) (-151.8261, 93.8192) (-151.6624, 93.5356) (-151.4792, 93.5356) knots 0 0 0 1 2 2 2
  spline S171 degree 2 poles (-151.4792, 93.5356) (-151.3723, 93.5356) (-151.1713, 93.6312) (-151.0821, 93.7058) knots 0 0 0 1 2 2 2
  line L184 (-151.0821, 93.7058) -> (-151.0821, 94.5583)
  spline S172 degree 2 poles (-151.0821, 94.5583) (-151.181, 94.6053) (-151.322, 94.6409) (-151.4128, 94.6409) knots 0 0 0 1 2 2 2
  spline S173 degree 2 poles (-151.4128, 94.6409) (-151.6089, 94.6409) (-151.8261, 94.3524) (-151.8261, 94.0769) knots 0 0 0 1 2 2 2
  spline S174 degree 2 poles (-153.0011, 94.8727) (-152.6413, 94.8727) (-152.2458, 94.4691) (-152.2458, 94.0964) knots 0 0 0 1 2 2 2
  spline S175 degree 2 poles (-152.2458, 94.0964) (-152.2458, 93.7301) (-152.63, 93.2957) (-152.9395, 93.2957) knots 0 0 0 1 2 2 2
  spline S176 degree 2 poles (-152.9395, 93.2957) (-153.0789, 93.2957) (-153.2945, 93.3767) (-153.3739, 93.4626) knots 0 0 0 1 2 2 2
  spline S177 degree 2 poles (-153.3739, 93.4626) (-153.4549, 93.5485) (-153.5408, 93.7965) (-153.5408, 93.9764) knots 0 0 0 1 2 2 2
  line L185 (-153.5408, 93.9764) -> (-153.5408, 94.1142)
  line L186 (-153.5408, 94.1142) -> (-152.5019, 94.1142)
  spline S178 degree 2 poles (-152.5019, 94.1142) (-152.5019, 94.3751) (-152.7645, 94.6523) (-152.9979, 94.6523) knots 0 0 0 1 2 2 2
  spline S179 degree 2 poles (-152.9979, 94.6523) (-153.0805, 94.6523) (-153.241, 94.615) (-153.3058, 94.5858) knots 0 0 0 1 2 2 2
  spline S180 degree 2 poles (-153.3058, 94.5858) (-153.3739, 94.5534) (-153.4679, 94.4967) (-153.4987, 94.4707) knots 0 0 0 1 2 2 2
  line L187 (-153.4987, 94.4707) -> (-153.5133, 94.4707)
  line L188 (-153.5133, 94.4707) -> (-153.5133, 94.7463)
  spline S181 degree 2 poles (-153.5133, 94.7463) (-153.4695, 94.7641) (-153.3366, 94.816) (-153.2847, 94.8306) knots 0 0 0 1 2 2 2
  spline S182 degree 2 poles (-153.2847, 94.8306) (-153.2118, 94.8516) (-153.0919, 94.8727) (-153.0011, 94.8727) knots 0 0 0 1 2 2 2
  spline S183 degree 2 poles (-153.2945, 93.9213) (-153.2912, 93.8192) (-153.2491, 93.6701) (-153.2086, 93.6199) knots 0 0 0 1 2 2 2
  spline S184 degree 2 poles (-153.2086, 93.6199) (-153.1648, 93.5631) (-153.027, 93.5032) (-152.9249, 93.5032) knots 0 0 0 1 2 2 2
  spline S185 degree 2 poles (-152.9249, 93.5032) (-152.8244, 93.5032) (-152.6834, 93.5631) (-152.6251, 93.6215) knots 0 0 0 1 2 2 2
  spline S186 degree 2 poles (-152.6251, 93.6215) (-152.5684, 93.6814) (-152.51, 93.8257) (-152.5019, 93.9213) knots 0 0 0 1 2 2 2
  line L189 (-152.5019, 93.9213) -> (-153.2945, 93.9213)
  line L190 (-154.5927, 93.6085) -> (-154.5797, 93.6085)
  spline S187 degree 2 poles (-154.5797, 93.6085) (-154.5505, 93.6004) (-154.4873, 93.5972) (-154.4436, 93.5972) knots 0 0 0 1 2 2 2
  spline S188 degree 2 poles (-154.4436, 93.5972) (-154.3415, 93.5972) (-154.1405, 93.6863) (-154.0497, 93.7738) knots 0 0 0 1 2 2 2
  line L191 (-154.0497, 93.7738) -> (-154.0497, 94.8387)
  line L192 (-154.0497, 94.8387) -> (-153.7969, 94.8387)
  line L193 (-153.7969, 94.8387) -> (-153.7969, 93.3378)
  line L194 (-153.7969, 93.3378) -> (-154.0497, 93.3378)
  line L195 (-154.0497, 93.3378) -> (-154.0497, 93.5615)
  spline S189 degree 2 poles (-154.0497, 93.5615) (-154.1875, 93.4383) (-154.3933, 93.3378) (-154.4906, 93.3378) knots 0 0 0 1 2 2 2
  spline S190 degree 2 poles (-154.4906, 93.3378) (-154.5295, 93.3378) (-154.5684, 93.3411) (-154.5927, 93.3459) knots 0 0 0 1 2 2 2
  line L196 (-154.5927, 93.3459) -> (-154.5927, 93.6085)
  spline S191 degree 2 poles (-155.194, 94.8743) (-155.0432, 94.8743) (-154.7823, 94.7933) (-154.6964, 94.7479) knots 0 0 0 1 2 2 2
  line L197 (-154.6964, 94.7479) -> (-154.6964, 94.4643)
  line L198 (-154.6964, 94.4643) -> (-154.7094, 94.4643)
  spline S192 degree 2 poles (-154.7094, 94.4643) (-154.7418, 94.4902) (-154.8293, 94.5518) (-154.9022, 94.5858) knots 0 0 0 1 2 2 2
  spline S193 degree 2 poles (-154.9022, 94.5858) (-154.9655, 94.6166) (-155.121, 94.662) (-155.2037, 94.662) knots 0 0 0 1 2 2 2
  spline S194 degree 2 poles (-155.2037, 94.662) (-155.2637, 94.662) (-155.4014, 94.6344) (-155.4338, 94.6118) knots 0 0 0 1 2 2 2
  spline S195 degree 2 poles (-155.4338, 94.6118) (-155.4809, 94.581) (-155.523, 94.5113) (-155.523, 94.44) knots 0 0 0 1 2 2 2
  spline S196 degree 2 poles (-155.523, 94.44) (-155.523, 94.3508) (-155.4257, 94.2584) (-155.3009, 94.2276) knots 0 0 0 1 2 2 2
  spline S197 degree 2 poles (-155.3009, 94.2276) (-155.2523, 94.2163) (-155.0967, 94.1839) (-155.0303, 94.166) knots 0 0 0 1 2 2 2
  spline S198 degree 2 poles (-155.0303, 94.166) (-154.8585, 94.1158) (-154.7029, 93.9083) (-154.7029, 93.7609) knots 0 0 0 1 2 2 2
  spline S199 degree 2 poles (-154.7029, 93.7609) (-154.7029, 93.5566) (-155.0092, 93.3022) (-155.262, 93.3022) knots 0 0 0 1 2 2 2
  spline S200 degree 2 poles (-155.262, 93.3022) (-155.3868, 93.3022) (-155.6397, 93.3638) (-155.7256, 93.4108) knots 0 0 0 1 2 2 2
  line L199 (-155.7256, 93.4108) -> (-155.7256, 93.6814)
  line L200 (-155.7256, 93.6814) -> (-155.7126, 93.6814)
  spline S201 degree 2 poles (-155.7126, 93.6814) (-155.6154, 93.6036) (-155.3787, 93.5145) (-155.2572, 93.5145) knots 0 0 0 1 2 2 2
  spline S202 degree 2 poles (-155.2572, 93.5145) (-155.1324, 93.5145) (-154.9606, 93.6199) (-154.9606, 93.7252) knots 0 0 0 1 2 2 2
  spline S203 degree 2 poles (-154.9606, 93.7252) (-154.9606, 93.8208) (-155.0627, 93.9132) (-155.1762, 93.9424) knots 0 0 0 1 2 2 2
  spline S204 degree 2 poles (-155.1762, 93.9424) (-155.2313, 93.957) (-155.3706, 93.9861) (-155.4468, 94.004) knots 0 0 0 1 2 2 2
  spline S205 degree 2 poles (-155.4468, 94.004) (-155.6121, 94.0461) (-155.7807, 94.239) (-155.7807, 94.4059) knots 0 0 0 1 2 2 2
  spline S206 degree 2 poles (-155.7807, 94.4059) (-155.7807, 94.5032) (-155.7045, 94.675) (-155.63, 94.7382) knots 0 0 0 1 2 2 2
  spline S207 degree 2 poles (-155.63, 94.7382) (-155.5505, 94.8046) (-155.3479, 94.8743) (-155.194, 94.8743) knots 0 0 0 1 2 2 2
  spline S208 degree 2 poles (-157.2734, 94.0477) (-157.2734, 94.4237) (-156.9152, 94.8678) (-156.6413, 94.8678) knots 0 0 0 1 2 2 2
  spline S209 degree 2 poles (-156.6413, 94.8678) (-156.5295, 94.8678) (-156.3577, 94.816) (-156.2685, 94.7625) knots 0 0 0 1 2 2 2
  line L201 (-156.2685, 94.7625) -> (-156.2685, 95.3913)
  line L202 (-156.2685, 95.3913) -> (-156.0157, 95.3913)
  line L203 (-156.0157, 95.3913) -> (-156.0157, 93.3378)
  line L204 (-156.0157, 93.3378) -> (-156.2685, 93.3378)
  line L205 (-156.2685, 93.3378) -> (-156.2685, 93.4951)
  spline S210 degree 2 poles (-156.2685, 93.4951) (-156.3625, 93.4092) (-156.5927, 93.2957) (-156.7272, 93.2957) knots 0 0 0 1 2 2 2
  spline S211 degree 2 poles (-156.7272, 93.2957) (-156.9849, 93.2957) (-157.2734, 93.7041) (-157.2734, 94.0477) knots 0 0 0 1 2 2 2
  spline S212 degree 2 poles (-157.0125, 94.0769) (-157.0125, 93.8192) (-156.8488, 93.5356) (-156.6656, 93.5356) knots 0 0 0 1 2 2 2
  spline S213 degree 2 poles (-156.6656, 93.5356) (-156.5586, 93.5356) (-156.3577, 93.6312) (-156.2685, 93.7058) knots 0 0 0 1 2 2 2
  line L206 (-156.2685, 93.7058) -> (-156.2685, 94.5583)
  spline S214 degree 2 poles (-156.2685, 94.5583) (-156.3674, 94.6053) (-156.5084, 94.6409) (-156.5992, 94.6409) knots 0 0 0 1 2 2 2
  spline S215 degree 2 poles (-156.5992, 94.6409) (-156.7953, 94.6409) (-157.0125, 94.3524) (-157.0125, 94.0769) knots 0 0 0 1 2 2 2
  spline S216 degree 2 poles (-158.1875, 94.8727) (-157.8277, 94.8727) (-157.4322, 94.4691) (-157.4322, 94.0964) knots 0 0 0 1 2 2 2
  spline S217 degree 2 poles (-157.4322, 94.0964) (-157.4322, 93.7301) (-157.8163, 93.2957) (-158.1259, 93.2957) knots 0 0 0 1 2 2 2
  spline S218 degree 2 poles (-158.1259, 93.2957) (-158.2653, 93.2957) (-158.4809, 93.3767) (-158.5603, 93.4626) knots 0 0 0 1 2 2 2
  spline S219 degree 2 poles (-158.5603, 93.4626) (-158.6413, 93.5485) (-158.7272, 93.7965) (-158.7272, 93.9764) knots 0 0 0 1 2 2 2
  line L207 (-158.7272, 93.9764) -> (-158.7272, 94.1142)
  line L208 (-158.7272, 94.1142) -> (-157.6883, 94.1142)
  spline S220 degree 2 poles (-157.6883, 94.1142) (-157.6883, 94.3751) (-157.9509, 94.6523) (-158.1843, 94.6523) knots 0 0 0 1 2 2 2
  spline S221 degree 2 poles (-158.1843, 94.6523) (-158.2669, 94.6523) (-158.4274, 94.615) (-158.4922, 94.5858) knots 0 0 0 1 2 2 2
  spline S222 degree 2 poles (-158.4922, 94.5858) (-158.5603, 94.5534) (-158.6543, 94.4967) (-158.6851, 94.4707) knots 0 0 0 1 2 2 2
  line L209 (-158.6851, 94.4707) -> (-158.6997, 94.4707)
  line L210 (-158.6997, 94.4707) -> (-158.6997, 94.7463)
  spline S223 degree 2 poles (-158.6997, 94.7463) (-158.6559, 94.7641) (-158.523, 94.816) (-158.4711, 94.8306) knots 0 0 0 1 2 2 2
  spline S224 degree 2 poles (-158.4711, 94.8306) (-158.3982, 94.8516) (-158.2783, 94.8727) (-158.1875, 94.8727) knots 0 0 0 1 2 2 2
  spline S225 degree 2 poles (-158.4809, 93.9213) (-158.4776, 93.8192) (-158.4355, 93.6701) (-158.395, 93.6199) knots 0 0 0 1 2 2 2
  spline S226 degree 2 poles (-158.395, 93.6199) (-158.3512, 93.5631) (-158.2134, 93.5032) (-158.1113, 93.5032) knots 0 0 0 1 2 2 2
  spline S227 degree 2 poles (-158.1113, 93.5032) (-158.0108, 93.5032) (-157.8698, 93.5631) (-157.8115, 93.6215) knots 0 0 0 1 2 2 2
  spline S228 degree 2 poles (-157.8115, 93.6215) (-157.7548, 93.6814) (-157.6964, 93.8257) (-157.6883, 93.9213) knots 0 0 0 1 2 2 2
  line L211 (-157.6883, 93.9213) -> (-158.4809, 93.9213)
  spline S229 degree 2 poles (-159.5797, 94.8727) (-159.4241, 94.8727) (-159.1664, 94.7771) (-159.074, 94.6798) knots 0 0 0 1 2 2 2
  spline S230 degree 2 poles (-159.074, 94.6798) (-158.9817, 94.5842) (-158.8796, 94.2892) (-158.8796, 94.0915) knots 0 0 0 1 2 2 2
  spline S231 degree 2 poles (-158.8796, 94.0915) (-158.8796, 93.8938) (-158.9849, 93.6053) (-159.074, 93.508) knots 0 0 0 1 2 2 2
  spline S232 degree 2 poles (-159.074, 93.508) (-159.1632, 93.4092) (-159.4274, 93.3038) (-159.5797, 93.3038) knots 0 0 0 1 2 2 2
  spline S233 degree 2 poles (-159.5797, 93.3038) (-159.7029, 93.3038) (-159.933, 93.3735) (-160.0222, 93.4189) knots 0 0 0 1 2 2 2
  line L212 (-160.0222, 93.4189) -> (-160.0222, 93.7025)
  line L213 (-160.0222, 93.7025) -> (-160.0076, 93.7025)
  spline S234 degree 2 poles (-160.0076, 93.7025) (-159.98, 93.6798) (-159.8958, 93.6215) (-159.8358, 93.5907) knots 0 0 0 1 2 2 2
  spline S235 degree 2 poles (-159.8358, 93.5907) (-159.7823, 93.5647) (-159.6397, 93.5242) (-159.5749, 93.5242) knots 0 0 0 1 2 2 2
  spline S236 degree 2 poles (-159.5749, 93.5242) (-159.3787, 93.5242) (-159.1405, 93.8208) (-159.1405, 94.0915) knots 0 0 0 1 2 2 2
  spline S237 degree 2 poles (-159.1405, 94.0915) (-159.1405, 94.3557) (-159.3706, 94.6523) (-159.5749, 94.6523) knots 0 0 0 1 2 2 2
  spline S238 degree 2 poles (-159.5749, 94.6523) (-159.698, 94.6523) (-159.9217, 94.5502) (-160.0076, 94.4707) knots 0 0 0 1 2 2 2
  line L214 (-160.0076, 94.4707) -> (-160.0222, 94.4707)
  line L215 (-160.0222, 94.4707) -> (-160.0222, 94.7544)
  spline S239 degree 2 poles (-160.0222, 94.7544) (-159.9849, 94.7722) (-159.8715, 94.8224) (-159.8261, 94.8338) knots 0 0 0 1 2 2 2
  spline S240 degree 2 poles (-159.8261, 94.8338) (-159.7612, 94.8532) (-159.6591, 94.8727) (-159.5797, 94.8727) knots 0 0 0 1 2 2 2
  spline S241 degree 2 poles (-160.7061, 94.8678) (-160.5003, 94.8678) (-160.2685, 94.6328) (-160.2685, 94.3784) knots 0 0 0 1 2 2 2
  line L216 (-160.2685, 94.3784) -> (-160.2685, 93.5469)
  line L217 (-160.2685, 93.5469) -> (-160.0984, 93.5469)
  line L218 (-160.0984, 93.5469) -> (-160.0984, 93.3378)
  line L219 (-160.0984, 93.3378) -> (-160.2685, 93.3378)
  line L220 (-160.2685, 93.3378) -> (-160.2685, 92.9067)
  line L221 (-160.2685, 92.9067) -> (-160.5214, 92.9067)
  line L222 (-160.5214, 92.9067) -> (-160.5214, 93.3378)
  line L223 (-160.5214, 93.3378) -> (-160.9865, 93.3378)
  line L224 (-160.9865, 93.3378) -> (-160.9865, 93.5469)
  line L225 (-160.9865, 93.5469) -> (-160.5214, 93.5469)
  line L226 (-160.5214, 93.5469) -> (-160.5214, 94.2617)
  spline S242 degree 2 poles (-160.5214, 94.2617) (-160.5214, 94.3751) (-160.5295, 94.4999) (-160.557, 94.5534) knots 0 0 0 1 2 2 2
  spline S243 degree 2 poles (-160.557, 94.5534) (-160.5797, 94.6004) (-160.6818, 94.6474) (-160.7693, 94.6474) knots 0 0 0 1 2 2 2
  spline S244 degree 2 poles (-160.7693, 94.6474) (-160.8309, 94.6474) (-160.946, 94.6101) (-160.9719, 94.5988) knots 0 0 0 1 2 2 2
  line L227 (-160.9719, 94.5988) -> (-160.9865, 94.5988)
  line L228 (-160.9865, 94.5988) -> (-160.9865, 94.8257)
  spline S245 degree 2 poles (-160.9865, 94.8257) (-160.9152, 94.8451) (-160.7693, 94.8678) (-160.7061, 94.8678) knots 0 0 0 1 2 2 2
  line L229 (-161.9687, 93.6085) -> (-161.9557, 93.6085)
  spline S246 degree 2 poles (-161.9557, 93.6085) (-161.9266, 93.6004) (-161.8633, 93.5972) (-161.8196, 93.5972) knots 0 0 0 1 2 2 2
  spline S247 degree 2 poles (-161.8196, 93.5972) (-161.7175, 93.5972) (-161.5165, 93.6863) (-161.4257, 93.7738) knots 0 0 0 1 2 2 2
  line L230 (-161.4257, 93.7738) -> (-161.4257, 94.8387)
  line L231 (-161.4257, 94.8387) -> (-161.1729, 94.8387)
  line L232 (-161.1729, 94.8387) -> (-161.1729, 93.3378)
  line L233 (-161.1729, 93.3378) -> (-161.4257, 93.3378)
  line L234 (-161.4257, 93.3378) -> (-161.4257, 93.5615)
  spline S248 degree 2 poles (-161.4257, 93.5615) (-161.5635, 93.4383) (-161.7693, 93.3378) (-161.8666, 93.3378) knots 0 0 0 1 2 2 2
  spline S249 degree 2 poles (-161.8666, 93.3378) (-161.9055, 93.3378) (-161.9444, 93.3411) (-161.9687, 93.3459) knots 0 0 0 1 2 2 2
  line L235 (-161.9687, 93.3459) -> (-161.9687, 93.6085)
  spline S250 degree 2 poles (-163.0011, 94.6798) (-162.9703, 94.7025) (-162.8666, 94.7835) (-162.818, 94.8079) knots 0 0 0 1 2 2 2
  spline S251 degree 2 poles (-162.818, 94.8079) (-162.7515, 94.8435) (-162.6267, 94.8808) (-162.5133, 94.8808) knots 0 0 0 1 2 2 2
  spline S252 degree 2 poles (-162.5133, 94.8808) (-162.4209, 94.8808) (-162.2539, 94.8111) (-162.1907, 94.7479) knots 0 0 0 1 2 2 2
  spline S253 degree 2 poles (-162.1907, 94.7479) (-162.1308, 94.6863) (-162.0578, 94.5048) (-162.0578, 94.4043) knots 0 0 0 1 2 2 2
  spline S254 degree 2 poles (-162.0578, 94.4043) (-162.0578, 94.2487) (-162.1891, 94.0283) (-162.3317, 93.9651) knots 0 0 0 1 2 2 2
  spline S255 degree 2 poles (-162.3317, 93.9651) (-162.4582, 93.9067) (-162.8018, 93.863) (-163.0011, 93.8516) knots 0 0 0 1 2 2 2
  line L236 (-163.0011, 93.8516) -> (-163.0011, 93.803)
  spline S256 degree 2 poles (-163.0011, 93.803) (-163.0011, 93.7155) (-162.9476, 93.6069) (-162.899, 93.5761) knots 0 0 0 1 2 2 2
  spline S257 degree 2 poles (-162.899, 93.5761) (-162.8504, 93.5453) (-162.711, 93.5259) (-162.6364, 93.5259) knots 0 0 0 1 2 2 2
  spline S258 degree 2 poles (-162.6364, 93.5259) (-162.5489, 93.5259) (-162.3123, 93.5777) (-162.194, 93.628) knots 0 0 0 1 2 2 2
  line L237 (-162.194, 93.628) -> (-162.1794, 93.628)
  line L238 (-162.1794, 93.628) -> (-162.1794, 93.3703)
  spline S259 degree 2 poles (-162.1794, 93.3703) (-162.2491, 93.3508) (-162.51, 93.3022) (-162.6381, 93.3022) knots 0 0 0 1 2 2 2
  spline S260 degree 2 poles (-162.6381, 93.3022) (-162.7937, 93.3022) (-163.006, 93.3508) (-163.0903, 93.414) knots 0 0 0 1 2 2 2
  spline S261 degree 2 poles (-163.0903, 93.414) (-163.1729, 93.4756) (-163.2539, 93.6717) (-163.2539, 93.8127) knots 0 0 0 1 2 2 2
  line L239 (-163.2539, 93.8127) -> (-163.2539, 94.8387)
  line L240 (-163.2539, 94.8387) -> (-163.0011, 94.8387)
  line L241 (-163.0011, 94.8387) -> (-163.0011, 94.6798)
  line L242 (-163.0011, 94.4691) -> (-163.0011, 94.0526)
  spline S262 degree 2 poles (-163.0011, 94.0526) (-162.9103, 94.0607) (-162.6364, 94.0882) (-162.5505, 94.1142) knots 0 0 0 1 2 2 2
  spline S263 degree 2 poles (-162.5505, 94.1142) (-162.4501, 94.145) (-162.3188, 94.273) (-162.3188, 94.3865) knots 0 0 0 1 2 2 2
  spline S264 degree 2 poles (-162.3188, 94.3865) (-162.3188, 94.5161) (-162.4646, 94.6474) (-162.604, 94.6474) knots 0 0 0 1 2 2 2
  spline S265 degree 2 poles (-162.604, 94.6474) (-162.7223, 94.6474) (-162.9168, 94.5453) (-163.0011, 94.4691) knots 0 0 0 1 2 2 2
  line L243 (-163.8666, 94.8387) -> (-163.6138, 94.8387)
  line L244 (-163.6138, 94.8387) -> (-163.6138, 92.7495)
  line L245 (-163.6138, 92.7495) -> (-163.8666, 92.7495)
  line L246 (-163.8666, 92.7495) -> (-163.8666, 94.8387)
  spline S266 degree 2 poles (-165.6932, 94.8727) (-165.5376, 94.8727) (-165.2799, 94.7771) (-165.1875, 94.6798) knots 0 0 0 1 2 2 2
  spline S267 degree 2 poles (-165.1875, 94.6798) (-165.0951, 94.5842) (-164.993, 94.2892) (-164.993, 94.0915) knots 0 0 0 1 2 2 2
  spline S268 degree 2 poles (-164.993, 94.0915) (-164.993, 93.8938) (-165.0984, 93.6053) (-165.1875, 93.508) knots 0 0 0 1 2 2 2
  spline S269 degree 2 poles (-165.1875, 93.508) (-165.2766, 93.4092) (-165.5408, 93.3038) (-165.6932, 93.3038) knots 0 0 0 1 2 2 2
  spline S270 degree 2 poles (-165.6932, 93.3038) (-165.8163, 93.3038) (-166.0465, 93.3735) (-166.1356, 93.4189) knots 0 0 0 1 2 2 2
  line L247 (-166.1356, 93.4189) -> (-166.1356, 93.7025)
  line L248 (-166.1356, 93.7025) -> (-166.121, 93.7025)
  spline S271 degree 2 poles (-166.121, 93.7025) (-166.0935, 93.6798) (-166.0092, 93.6215) (-165.9492, 93.5907) knots 0 0 0 1 2 2 2